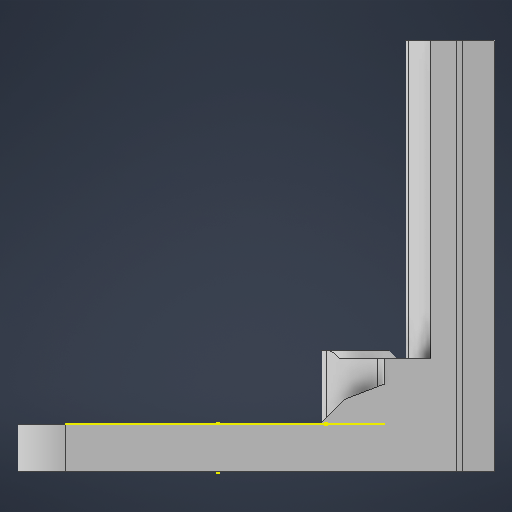
# Autodesk Inventor part: guideline
Saved by Autodesk Inventor 2026 (Build 300175000, 175)
## iProperties
Created: 2025-11-28
Part Number: guideline
Material: 一般
Document SubType Name: Modeling
Designer: numai
Density: 1 g/cm^3
Appearance: 既定
Author: numai
Autodesk Inventor part; units mm, degrees
ref_plane "YZ Plane" through (0, 0, 0) normal (1, 0, 0) x (0, 1, 0)
ref_plane "XZ Plane" through (0, 0, 0) normal (0, 1, 0) x (-1, 0, 0)
sketch "スケッチ1" plane through (0, 0, 0) normal (0, 0, 1) x (1, 0, 0)
  circle A0 centre (0, 0) radius 17.3 construction
  line L0 (0, 0) -> (0, 20.4) construction
  circle A1 centre (0, -17.3) radius 3 construction
  circle A2 centre (0, 0) radius 14.3 construction
  circle A3 centre (0, 0) radius 20.3 construction
  circle A4 centre (0, 17.3) radius 3 construction
  circle A5 centre (-8.65, 14.9822) radius 3 construction
  line L1 (-8.65, 14.9822) -> (0, 17.3) construction
  line L2 (-8.65, 14.9822) -> (0, 0) construction
  line L3 (-8.65, 14.9822) -> (8.65, 14.9822) construction
  line L4 (0, 0) -> (8.65, 14.9822) construction
  line L5 (0, 17.3) -> (8.65, 14.9822) construction
  circle A6 centre (8.65, 14.9822) radius 3 construction
  arc A7 (-33.421, 8.3449) -> (33.421, 8.3449) centre (0, 17.3) ccw construction
  line L6 (-8.65, 14.9822) -> (-33.421, 8.3449) construction
  line L7 (8.65, 14.9822) -> (33.421, 8.3449) construction
  arc A8 (-8.65, 14.9822) -> (8.65, 14.9822) centre (0, 17.3) ccw construction
  circle A9 centre (0, 8.3449) radius 3 construction
  line L8 (3, 8.3449) -> (3, -17.3) construction
  line L9 (-3, 8.3449) -> (-3, -17.3) construction
  line L10 (0, -20.3) -> (0, -26) construction
  circle A10 centre (0, 17.3) radius 15.3358 construction
  circle A11 centre (0, 17.3) radius 7 construction
  line L11 (-4.9497, 22.2497) -> (4.9497, 22.2497) construction
  line L12 (4.9497, 22.2497) -> (4.9497, 12.3503) construction
  line L13 (4.9497, 12.3503) -> (-4.9497, 12.3503) construction
  line L14 (-4.9497, 12.3503) -> (-4.9497, 22.2497) construction
  circle A12 centre (0, 17.3) radius 1.6
  line L15 (0, 8.3449) -> (0, -17.7) construction
  arc A13 (3, 8.3449) -> (-3, 8.3449) centre (0, 8.3449) ccw
  line L16 (0, 17.3) -> (0, -17.7) construction
  line L17 (-7.5, 17.3) -> (-7.5, -17.7) construction
  line L18 (7.5, -17.7) -> (7.5, 17.3) construction
  arc A14 (7.5, 17.3) -> (-7.5, 17.3) centre (0, 17.3) ccw construction
  arc A15 (-7.5, -17.7) -> (7.5, -17.7) centre (0, -17.7) ccw
  circle A16 centre (4.9497, 22.2497) radius 1.25
  circle A17 centre (-4.9497, 22.2497) radius 1.25
  circle A18 centre (-4.9497, 12.3503) radius 1.25
  circle A19 centre (4.9497, 12.3503) radius 1.25
  circle A20 centre (0, 17.3) radius 20 construction
  circle A21 centre (0, -17.7) radius 35 construction
  arc A22 (15.3498, 21.9312) -> (-15.3498, 21.9312) centre (0, -17.7) ccw construction
  line L19 (17, 34.8) -> (-17, 34.8)
  line L20 (17, 34.8) -> (17, 26.8) construction
  line L21 (-17, 34.8) -> (-17, 26.8) construction
  line L22 (17, 26.8) -> (-17, 26.8) construction
  line L23 (17, 30.8) -> (-17, 30.8) construction
  line L24 (-13, 26.8) -> (-13, 34.8) construction
  line L25 (13, 26.8) -> (13, 34.8) construction
  circle A23 centre (13, 30.8) radius 1.25
  circle A24 centre (0, 30.8) radius 1.25
  circle A25 centre (-13, 30.8) radius 1.25
  arc A26 (-3, -17.7) -> (3, -17.7) centre (0, -17.7) ccw
  line L26 (-3, -17.7) -> (-3, 8.3449)
  line L27 (3, 8.3449) -> (3, -17.7)
  circle A27 centre (-13, 30.8) radius 4 construction
  circle A28 centre (13, 30.8) radius 4 construction
  line L28 (-16.9264, 30.0362) -> (-7.362, -19.1321)
  line L29 (7.362, -19.1321) -> (16.9264, 30.0362)
  line L30 (-17, 34.8) -> (-17, 30.8)
  arc A29 (-17, 30.8) -> (-16.9264, 30.0362) centre (-13, 30.8) ccw
  arc A30 (16.9264, 30.0362) -> (17, 30.8) centre (13, 30.8) ccw
  line L31 (17, 30.8) -> (17, 34.8)
  point P0 (-5.7522, 15.7587)
  point P1 (-2.8978, 16.5235)
  point P2 (0, -4.6776)
  point P3 (0, -0.2)
  point P4 (0, 24.8)
  point P5 (0, 10.2)
  point P6 (0, -17.3)
  point P7 (0, 34.8)
  dimension "d0" = 34.6
  dimension "d2" = 6
  dimension "d4" = 2.9551
  dimension "d5" = 150
  dimension "d8" = 14
  dimension "d11" = 3.2
  dimension "d14" = 2.5
  dimension "d15" = 17.3
  dimension "d16" = 40
  dimension "d17" = 10.2
  dimension "d18" = 17.5
  dimension "d19" = 8
  dimension "d20" = 4
  dimension "d21" = 4
  dimension "d22" = 4
  dimension "d23" = 2.5
  dimension "d40" = 0.4
  dimension "d41" = 4.5
  dimension "d44" = 26
  constraints: 70 end point, 39 point on circle, 27 centre point, 20 coincident, 17 tangent, 12 point on line, 9 midpoint, 7 equal radius, 7 vertical, 6 perpendicular, 5 horizontal, 4 vertical alignment, 3 parallel, 1 collinear, 1 concentric, 14 other
  measures "d0" diameter of A0
  measures "d2" diameter of A1
  measures "d4" distance of point (-5.752, 15.759) point (-2.898, 16.524)
  measures "d5" angle of L5 L1
  measures "d8" diameter of A11
  measures "d11" diameter of A12
  measures "d14" diameter of A16
  measures "d15" distance of L1.end point (0, 0)
  measures "d16" diameter of A20
  measures "d17" distance of point (0, 10.2) point (0, 0)
  measures "d18" distance from line of L19 L1.end
  measures "d19" distance between parallel lines of L19 L22
  measures "d20" distance between parallel lines of L19 L23
  measures "d21" distance between parallel lines of L21 L24
  measures "d22" distance between parallel lines of L25 L20
  measures "d23" diameter of A23
  measures "d40" distance of point (0, -17.3) A26.centre
  measures "d41" radial gap between concentric circles of A26 A15
  measures "d44" distance of A28.centre A25.centre
extrude "押し出し1" add sketch "スケッチ1" along normal blind 4 contours L28 A29 L30 L19 L31 A30 L29 A15 | A16 | A17 | A18 | A19
sketch "スケッチ2" plane through (0, 0, 4) normal (0, 0, 1) x (1, 0, 0)
  arc A0 (-7.362, -19.1321) -> (7.362, -19.1321) centre (0, -17.7) ccw projected
  line L0 (17, 34.8) -> (-17, 34.8) projected
  arc A1 (3, 8.3449) -> (-3, 8.3449) centre (0, 8.3449) ccw projected
  circle A2 centre (0, 17.3) radius 1.6 projected
  circle A3 centre (-13, 30.8) radius 1.25 projected
  circle A4 centre (0, 30.8) radius 1.25 projected
  circle A5 centre (13, 30.8) radius 1.25 projected
  circle A6 centre (0, 17.3) radius 10
  circle A7 centre (0, 17.3) radius 4.25
  line L1 (0, 17.3) -> (0, 34.8) construction
  line L2 (19.8551, 26.8) -> (-19.8551, 26.8)
  line L3 (-16.9264, 30.0362) -> (-7.362, -19.1321) projected
  line L4 (7.362, -19.1321) -> (16.9264, 30.0362) projected
  arc A8 (16.9264, 30.0362) -> (17, 30.8) centre (13, 30.8) ccw projected
  line L5 (17, 30.8) -> (17, 34.8) projected
  line L6 (-17, 34.8) -> (-17, 30.8) projected
  arc A9 (-17, 30.8) -> (-16.9264, 30.0362) centre (-13, 30.8) ccw projected
  line L7 (-3, -17.7) -> (-3, 8.3449) projected
  line L8 (3, 8.3449) -> (3, -17.7) projected
  arc A10 (-3, -17.7) -> (3, -17.7) centre (0, -17.7) ccw projected
  circle A11 centre (0, 17.3) radius 17 construction
  circle A12 centre (16.5925, 13.6) radius 7.5 construction
  line L9 (2.1986, 13.6629) -> (12.7126, 20.0185)
  line L10 (-2.1986, 13.6629) -> (-12.7126, 20.0185)
  arc A13 (15.1613, 20.9622) -> (12.7126, 20.0185) centre (16.5925, 13.6) ccw
  arc A14 (-12.7126, 20.0185) -> (-15.1613, 20.9622) centre (-16.5925, 13.6) ccw
  point P0 (0, 0)
  point P1 (6.8841, 24.5532)
  point P2 (16.2935, 29.35)
  point P3 (-2.1986, 13.6629)
  point P4 (-15.1613, 20.9622)
  point P5 (16.2969, 26.8)
  point P6 (-16.2969, 26.8)
  dimension "d24" = 20
  dimension "d25" = 8.5
  dimension "d42" = 34
  dimension "d29" = 8
  dimension "d43" = 15
  dimension "d46" = 13.2
  constraints: 8 end point, 6 point on circle, 4 coincident, 4 symmetric about line, 3 centre point, 1 midpoint, 1 parallel, 1 point on line, 1 tangent, 11 other
  measures "d29" distance between parallel lines of L2 L0
  measures "d43" diameter of A12
  measures "d46" distance from line of L2 A12.centre
extrude "押し出し2" add sketch "スケッチ2" along normal blind 11.3 contours L3 L2 A6 L10 A14 | A13 L9 A6 L2 L4 | L2 A6 L9 A7 L10 | A7
sketch "スケッチ3" plane through (0, 0, 15.3) normal (0, 0, 1) x (1, 0, 0)
  arc A0 (-2.1986, 13.6629) -> (2.1986, 13.6629) centre (0, 17.3) ccw projected
  circle A1 centre (0, 17.3) radius 1.6 projected
  circle A2 centre (0, 17.3) radius 4.25
  line L0 (2.1986, 13.6629) -> (12.7126, 20.0185) projected
  arc A3 (15.1613, 20.9622) -> (12.7126, 20.0185) centre (16.5925, 13.6) ccw projected
  line L1 (15.1613, 20.9622) -> (16.2969, 26.8) projected
  line L2 (16.2969, 26.8) -> (-16.2969, 26.8) projected
  line L3 (-16.2969, 26.8) -> (-15.1613, 20.9622) projected
  arc A4 (-12.7126, 20.0185) -> (-15.1613, 20.9622) centre (-16.5925, 13.6) ccw projected
  line L4 (-12.7126, 20.0185) -> (-2.1986, 13.6629) projected
  point P0 (0, 0)
  point P1 (2.1986, 13.6629)
  constraints: 1 centre point, 1 coincident, 1 concentric
extrude "押し出し3" cut sketch "スケッチ3" against normal blind 1 contours L4 A4 L3 L2 L1 A3 L0 A2
sketch "スケッチ4" plane through (0, 0, 4) normal (0, 0, 1) x (1, 0, 0)
  line L0 (17, 34.8) -> (-17, 34.8) projected
  circle A0 centre (-13, 30.8) radius 1.25 projected
  circle A1 centre (0, 30.8) radius 1.25 projected
  circle A2 centre (13, 30.8) radius 1.25 projected
  line L1 (-16.9264, 30.0362) -> (-16.2969, 26.8) projected
  arc A3 (-7.362, -19.1321) -> (7.362, -19.1321) centre (0, -17.7) ccw projected
  line L2 (7.362, -19.1321) -> (15.1613, 20.9622) projected
  arc A4 (16.9264, 30.0362) -> (17, 30.8) centre (13, 30.8) ccw projected
  line L3 (17, 30.8) -> (17, 34.8) projected
  line L4 (-17, 34.8) -> (-17, 30.8) projected
  arc A5 (-17, 30.8) -> (-16.9264, 30.0362) centre (-13, 30.8) ccw projected
  line L5 (-16.9264, 30.0362) -> (-7.362, -19.1321) projected
  line L6 (-16.7929, 29.35) -> (16.7929, 29.35)
  line L7 (-16.2969, 26.8) -> (16.2969, 26.8) projected
  line L8 (16.2969, 26.8) -> (16.9264, 30.0362) projected
  arc A6 (15.1613, 20.9622) -> (12.7126, 20.0185) centre (16.5925, 13.6) ccw projected
  line L9 (12.7126, 20.0185) -> (2.1986, 13.6629) projected
  arc A7 (-2.1986, 13.6629) -> (2.1986, 13.6629) centre (0, 17.3) ccw projected
  line L10 (-2.1986, 13.6629) -> (-12.7126, 20.0185) projected
  arc A8 (-12.7126, 20.0185) -> (-15.1613, 20.9622) centre (-16.5925, 13.6) ccw projected
  line L11 (-15.1613, 20.9622) -> (-7.362, -19.1321) projected
  point P0 (0, 0)
  point P1 (-16.2935, 29.35)
  point P2 (13.4899, 29.35)
  point P3 (12.5101, 29.35)
  point P4 (0.4899, 29.35)
  point P5 (-0.4899, 29.35)
  point P6 (-12.5101, 29.35)
  point P7 (-13.4899, 29.35)
  constraints: 3 point on line, 2 end point, 1 horizontal
extrude "押し出し4" add sketch "スケッチ4" along normal blind 50.3 contours L3 A4 L8 L6 L1 A5 L4 L0 | L8 L7 L1 L6
sketch "スケッチ5" plane through (0, 0, 0) normal (0, 0, -1) x (-1, 0, 0)
  point P0 (0, 0)
chamfer "面取り1" distance 1 angle 45 1 edges at (0, 21.55, 14.3)
sketch "スケッチ6" plane through (0, 0, 54.3) normal (0, 0, 1) x (1, 0, 0)
  line L0 (-16.2969, 26.8) -> (16.2969, 26.8) projected
  circle A0 centre (0, 30.8) radius 1.25 projected
  line L1 (-16.2969, 26.8) -> (16.2969, 26.8) projected
  line L2 (12.2644, 26.8) -> (0, 23.1904)
  line L3 (0, 23.1904) -> (-12.2644, 26.8)
  point P0 (0, 0)
  point P1 (12.2644, 26.8)
  dimension "d47" = 16.4
  dimension "d48" = 16.4
  dimension "d49" = 7.3
  constraints: 4 end point, 2 point on line, 1 vertical alignment
  measures "d47" angle of L0 L3
  measures "d48" angle of L0 L2
  measures "d49" distance from line of A0.centre L3
extrude "押し出し5" add sketch "スケッチ6" against normal up to surface (40 mm away) contours L0 L2 L3
fillet "フィレット2" radius 10 1 edges at (0, 23.1904, 34.3)
sketch "スケッチ7" plane through (0, 0, 54.3) normal (0, 0, 1) x (1, 0, 0)
  line L0 (-12.2644, 26.8) -> (-2.8234, 24.0214) projected
  line L1 (2.8234, 24.0214) -> (12.2644, 26.8) projected
  line L2 (-16.2969, 26.8) -> (-12.2644, 26.8) projected
  line L3 (12.2644, 26.8) -> (16.2969, 26.8) projected
  line L4 (-12.2644, 26.8) -> (-12.9222, 26.9936)
  line L5 (-12.9222, 26.9936) -> (-13.6549, 26.8)
  line L6 (-13.6549, 26.8) -> (-16.2969, 26.8)
  line L7 (17, 34.8) -> (-17, 34.8) projected
  circle A0 centre (-13, 30.8) radius 1.25 projected
  line L8 (0, 46.8) -> (0, -37.2) projected
  line L9 (12.2644, 26.8) -> (12.9222, 26.9936)
  line L10 (12.9222, 26.9936) -> (13.6549, 26.8)
  point P0 (0, 0)
  point P1 (13.6549, 26.8)
  point P2 (-13.6549, 26.8)
  dimension "d53" = 3.7
  dimension "d54" = 148.8
  constraints: 10 end point, 2 symmetric about line, 1 collinear, 1 parallel
  measures "d53" distance from line of A0.centre L5
  measures "d54" angle of L4 L5
extrude "押し出し6" cut sketch "スケッチ7" against normal up to surface (40 mm away) contours L5 L4 L2 | L9 L10 L3
sketch "スケッチ10" plane through (0, 0, 0) normal (0, 0, -1) x (-1, 0, 0)
  circle A0 centre (0, 17.3) radius 1.6 projected
  circle A1 centre (0, 17.3) radius 1.25
  point P0 (0, 0)
  dimension "d66" = 2.5
  constraints: 1 centre point, 1 coincident
  measures "d66" diameter of A1
extrude "押し出し9" add sketch "スケッチ10" against normal blind 12.8
sketch "スケッチ11" plane through (0, 0, 4) normal (0, 0, 1) x (1, 0, 0)
  point P0 (0, 0)
sketch "スケッチ12" plane through (0, 0, 4) normal (0, 0, 1) x (1, 0, 0)
  arc A0 (15.1613, 20.9622) -> (12.7126, 20.0185) centre (16.5925, 13.6) ccw projected
  line L0 (12.7126, 20.0185) -> (2.1986, 13.6629) projected
  arc A1 (-2.1986, 13.6629) -> (2.1986, 13.6629) centre (0, 17.3) ccw projected
  line L1 (-2.1986, 13.6629) -> (-12.7126, 20.0185) projected
  arc A2 (-12.7126, 20.0185) -> (-15.1613, 20.9622) centre (-16.5925, 13.6) ccw projected
  line L2 (-15.1613, 20.9622) -> (-7.362, -19.1321) projected
  arc A3 (-7.362, -19.1321) -> (7.362, -19.1321) centre (0, -17.7) ccw projected
  line L3 (7.362, -19.1321) -> (15.1613, 20.9622) projected
  line L4 (-3, -17.7) -> (-3, 8.3449) projected
  arc A4 (3, 8.3449) -> (-3, 8.3449) centre (0, 8.3449) ccw projected
  line L5 (3, 8.3449) -> (3, -17.7) projected
  arc A5 (-3, -17.7) -> (3, -17.7) centre (0, -17.7) ccw projected
  point P0 (0, 0)
extrude "押し出し10" add sketch "スケッチ12" along normal blind 2
sketch "スケッチ13" plane through (0, 0, 6) normal (0, 0, 1) x (1, 0, 0)
  arc A0 (15.1613, 20.9622) -> (12.7126, 20.0185) centre (16.5925, 13.6) ccw projected
  line L0 (2.1986, 13.6629) -> (12.7126, 20.0185) projected
  arc A1 (-2.1986, 13.6629) -> (2.1986, 13.6629) centre (0, 17.3) ccw projected
  line L1 (-12.7126, 20.0185) -> (-2.1986, 13.6629) projected
  arc A2 (-12.7126, 20.0185) -> (-15.1613, 20.9622) centre (-16.5925, 13.6) ccw projected
  line L2 (7.362, -19.1321) -> (15.1613, 20.9622) projected
  line L3 (-15.1613, 20.9622) -> (-7.362, -19.1321) projected
  point P0 (0, 0)
ref_plane "作業平面1" through (0, 13.05, 4) normal (0, 1, 0) x (1, 0, 0)
sketch "スケッチ14" plane through (0, 13.05, 4) normal (0, 1, 0) x (1, 0, 0)
  line L0 (15.1613, -2) -> (15.1613, -10.3) projected
  line L1 (-15.1613, -2) -> (-15.1613, -10.3) projected
  line L2 (12.7126, -10.3) -> (15.1613, -10.3) projected
  line L3 (-15.1613, -10.3) -> (-12.7126, -10.3) projected
  line L4 (-15.1613, -2) -> (-7.362, -2) projected
  line L5 (-7.362, -2) -> (7.362, -2) projected
  line L6 (15.1613, -2) -> (12.7126, -2) projected
  line L7 (2.1986, -2) -> (12.7126, -2) projected
  line L8 (15.1613, -7) -> (14.1613, -7)
  line L9 (14.1613, -7) -> (9.1613, -2)
  line L10 (-12.7126, -2) -> (-2.1986, -2) projected
  line L11 (-9.1613, -2) -> (-14.1613, -7)
  line L12 (-14.1613, -7) -> (-15.1613, -7)
  point P0 (0, 4)
  point P1 (-9.1613, -2)
  dimension "d76" = 45
  dimension "d77" = 45
  dimension "d78" = 5
  dimension "d79" = 1
  constraints: 8 end point, 6 point on line, 1 collinear, 1 horizontal
  measures "d76" angle of L7 L9
  measures "d77" angle of L10 L11
  measures "d78" distance from line of L8.start L6
  measures "d79" distance of L8.start L8.end
extrude "押し出し11" add sketch "スケッチ14" along normal blind 20
chamfer "面取り3" distance 3 angle 60 1 edges at (11.6613, 13.05, 8.5) measured on face at (12.0148, 13.05, 8.1464)
chamfer "面取り4" distance 3 angle 60 1 edges at (-11.6613, 13.05, 8.5) measured on face at (-12.0148, 13.05, 8.1464)
sketch "スケッチ15" plane through (0, 0, 0) normal (0, 0, -1) x (-1, 0, 0)
  line L0 (13.6222, 13.05) -> (15.1613, 13.05) projected
  line L1 (15.1613, 13.05) -> (15.1613, 20.9622) projected
  line L2 (15.1613, 20.9622) -> (13.6222, 13.05) projected
  line L3 (-13.6222, 13.05) -> (-15.1613, 20.9622) projected
  line L4 (-15.1613, 13.05) -> (-15.1613, 20.9622) projected
  line L5 (-15.1613, 13.05) -> (-13.6222, 13.05) projected
  point P0 (0, 0)
extrude "押し出し12" cut sketch "スケッチ15" against normal through all
chamfer "面取り5" distance 2.4 angle 45 2 edges at (-14.3517, 18.0129, 11) (14.3517, 18.0129, 11)
sketch "スケッチ16" plane through (-14.1771, 15.9029, 9.1026) normal (0.3410107, -0.278434, 0.8978787) x (0.9229232, 0.2807005, -0.2634767)
  line L0 (0, 0) -> (2.4235, 1.8104) projected
  ellipse E0 centre (-4.0161, -0.1571) end of major axis (-12.3488, 5.0696) minor radius 7.0847 (2.3887, 3.6768) -> (1.7675, 4.2962) ccw construction
  line L1 (2.3887, 3.6768) -> (5.3696, 0.4909) construction
  line L2 (2.4235, 1.8104) -> (3.4308, 2.563)
  line L3 (2.4235, 1.8104) -> (1.7675, 4.2962) projected
  line L4 (3.4308, 2.563) -> (3.8283, 2.8599)
  ellipse E1 centre (-2.9291, -1.6121) end of major axis (2.07, -8.304) minor radius 7.5 (1.7675, 4.2962) -> (0.1006, 5.4548) ccw projected
  line L5 (3.8283, 2.8599) -> (1.7675, 4.2962)
  point P0 (11.0188, -20.3507)
  constraints: 6 end point, 1 collinear, 1 point on line, 2 other
extrude "押し出し13" add sketch "スケッチ16" against normal blind 2
sketch "スケッチ18" plane through (-13.4039, 13.05, 6) normal (0.6123724, -0.5, 0.6123724) x (0.4743416, -0.3872983, -0.7905694)
  line L0 (-3.9246, 4.7459) -> (-3.9246, 6.0434) projected
  line L1 (-0.7835, 6.3165) -> (-3.9246, 4.7459) projected
  line L2 (-3.9246, 6.0434) -> (-1.9199, 7.291)
  line L3 (-1.9199, 7.291) -> (-0.7835, 6.3165)
  point P0 (16.1557, -1.6311)
  constraints: 4 end point
extrude "押し出し14" add sketch "スケッチ18" against normal blind 2
mirror "ミラー1" about plane through (0, 0, 0) normal (1, 0, 0) of "押し出し13", "押し出し14"
sketch "スケッチ8" plane through (0, 0, 15.3) normal (0, 0, 1) x (1, 0, 0)
  arc A0 (-1.8512, 13.7542) -> (1.8512, 13.7542) centre (0, 17.3) ccw projected
  arc A1 (1.8512, 13.7542) -> (-1.8512, 13.7542) centre (0, 17.3) ccw projected
  circle A2 centre (0, 17.3) radius 1.5 projected
  point P0 (0, 0)
equation "\"d20\" = 0.5 * d19"
equation "\"d21\" = d20"
equation "\"d22\" = d21"
equation "\"d48\" = d47"
